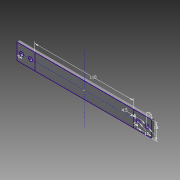
# Autodesk Inventor part: TopSliderBar
Saved by Autodesk Inventor 2014 SP1 (Build 180222100, 222)
## iProperties
Created: 2014-06-08
Part Number: TopSliderBar
Material: Generic
Document SubType Name: Modeling
Designer: Erin
Density: 1 g/cm^3
Appearance: Default
Author: Erin
Autodesk Inventor part; units mm, degrees
ref_plane "YZ Plane" through (0, 0, 0) normal (1, 0, 0) x (0, 1, 0)
ref_plane "XZ Plane" through (0, 0, 0) normal (0, 1, 0) x (-1, 0, 0)
ref_plane "XY Plane" through (0, 0, 0) normal (0, 0, 1) x (1, 0, 0)
sketch "Sketch1" plane through (0, 0, 0) normal (0, 1, 0) x (-1, 0, 0)
  line L0 (-75, 9) -> (0, 9)
  line L1 (75, 9) -> (75, -9)
  line L2 (75, -9) -> (0, -9)
  line L3 (-75, -9) -> (-75, 9)
  line L4 (-75, 0) -> (75, 0) construction
  circle A0 centre (-70, 0) radius 2.25
  circle A1 centre (-60, 0) radius 2.25
  line L5 (0, 9) -> (75, 9)
  line L6 (0, -9) -> (-75, -9)
  line L7 (-55, 9) -> (-55, -9)
  line L8 (0, 37.7423) -> (0, -37.3462) construction
  circle A2 centre (70, 0) radius 2.25
  circle A3 centre (60, 0) radius 2.25
  line L9 (55, 9) -> (55, -9)
  point P0 (0, 0)
  dimension "d1" = 18
  dimension "d2" = 4.5
  dimension "d3" = 4.5
  dimension "d4" = 5
  dimension "d5" = 15
  dimension "d17" = 5
  dimension "d18" = 110
  dimension "d19" = 5
  constraints: 20 end point, 6 parallel, 4 centre point, 4 perpendicular, 4 point on line, 4 symmetric about line, 2 horizontal, 2 midpoint, 1 horizontal alignment, 1 vertical, 1 vertical alignment, 2 other
  measures "d1" distance of L3.start L0.start
  measures "d2" diameter of A0
  measures "d3" diameter of A1
  measures "d4" distance from line of A0.centre L3
  measures "d5" distance from line of A1.centre L3
  measures "d17" distance from line of A1.centre L7
  measures "d18" distance between parallel lines of L9 L7
  measures "d19" distance from line of A2.centre L1
extrude "Extrusion1" add sketch "Sketch1" along normal blind 3
sketch "Sketch2" plane through (0, 3, 0) normal (0, 1, 0) x (1, 0, 0)
  line L0 (-50, 1.5) -> (50, 1.5)
  line L1 (50, 1.5) -> (50, -1.5)
  line L2 (50, -1.5) -> (-50, -1.5)
  line L3 (-50, -1.5) -> (-50, 1.5)
  point P0 (0, 0)
  point P1 (50, 0)
  point P2 (0, 1.5)
  dimension "d20" = 100
  dimension "d21" = 3
  constraints: 8 end point, 2 midpoint, 2 parallel, 1 horizontal, 1 horizontal alignment, 1 perpendicular, 1 vertical alignment
  measures "d20" distance of L0.start L0.end
  measures "d21" distance of L2.end L0.start
extrude "Extrusion3" add sketch "Sketch2" along normal blind 3
body "Solid1"
